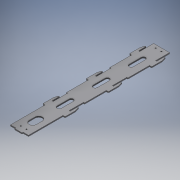
# Autodesk Inventor part: Camera mounting back
Saved by Autodesk Inventor 2017 (Build 210142000, 142)
## iProperties
Created: 2016-08-03
Part Number: Camera mounting back
Material: Generic
Document SubType Name: Modeling
Designer: Ali
Density: 1 g/cm^3
Appearance: Default
Author: Ali
Autodesk Inventor part; units mm, degrees
ref_plane "YZ Plane" through (0, 0, 0) normal (1, 0, 0) x (0, 1, 0)
ref_plane "XZ Plane" through (0, 0, 0) normal (0, 1, 0) x (-1, 0, 0)
ref_plane "XY Plane" through (0, 0, 0) normal (0, 0, 1) x (1, 0, 0)
sketch "Sketch1" plane through (0, 0, 0) normal (0, 0, 1) x (1, 0, 0)
  line L0 (-25, 0) -> (25, 0)
  line L1 (25, 0) -> (25, 394)
  line L2 (25, 394) -> (-25, 394)
  line L3 (-25, 394) -> (-25, 0)
  point P0 (0, 0)
  point P1 (0, 0)
  dimension "d0" = 394
  dimension "d1" = 50
  constraints: 8 end point, 3 perpendicular, 1 coincident, 1 horizontal, 1 midpoint
  measures "d0" distance of L0.end L1.end
  measures "d1" distance of L0.start L0.end
extrude "Extrusion1" add sketch "Sketch1" along normal blind 3
sketch "Sketch2" plane through (0, 0, 0) normal (0, 0, -1) x (-1, 0, 0)
  line L0 (-22, 334) -> (-25, 334)
  line L1 (-22, 374) -> (-25, 374)
  line L2 (-22, 374) -> (-22, 354)
  line L3 (-25, 334) -> (-25, 354)
  line L4 (-25, 0) -> (-25, 394) projected
  line L5 (-22, 354) -> (-25, 354)
  line L6 (-25, 0) -> (-25, 394) projected
  line L7 (-25, 394) -> (25, 394) projected
  line L8 (-25, 354) -> (-25, 374)
  line L9 (-22, 354) -> (-22, 334)
  line L10 (-22, 374) -> (-25, 374)
  line L11 (-25, 374) -> (-25, 394)
  line L12 (-25, 394) -> (-22, 394)
  line L13 (-22, 394) -> (-22, 374)
  point P0 (0, 0)
  dimension "d4" = 20
  dimension "d10" = 20
  dimension "d55" = 60
  dimension "d56" = 20
  constraints: 22 end point, 3 perpendicular, 3 point on line, 2 collinear, 2 parallel, 2 vertical, 1 horizontal
  measures "d4" distance between parallel lines of L1 L5
  measures "d10" distance of L12.end L1.start
  measures "d55" distance between parallel lines of L7 L0
  measures "d56" distance of L2.end L0.start
extrude "Extrusion2" cut sketch "Sketch2" against normal blind 3 contours L5 L4 L1 L2 | L1 L4 L7 L13
sketch "Sketch3" plane through (0, 0, 0) normal (0, 0, -1) x (-1, 0, 0)
  line L0 (-25, 0) -> (-25, 354) projected
  line L1 (-25, 354) -> (-31, 354)
  line L2 (-31, 354) -> (-31, 336)
  line L3 (-29, 334) -> (-25, 334)
  line L4 (-25, 334) -> (-25, 354)
  line L5 (-31, 354) -> (-25, 354)
  line L6 (-25, 354) -> (-25, 374)
  line L7 (-25, 374) -> (-28, 374)
  line L8 (-31, 364) -> (-31, 354)
  line L9 (-31, 364) -> (-28, 374)
  line L10 (-28, 374) -> (-31, 374) construction
  arc A0 (-31, 336) -> (-29, 334) centre (-29, 336) ccw
  point P0 (0, 0)
  point P1 (-31, 334)
  dimension "d11" = 20
  dimension "d12" = 20
  dimension "d13" = 6
  dimension "d16" = 2
  constraints: 20 end point, 5 parallel, 3 point on line, 2 horizontal, 2 perpendicular, 2 point on circle, 2 tangent, 1 centre point
  measures "d11" distance of L1.end point (-31, 334)
  measures "d12" distance of L10.end L1.end
  measures "d13" distance between parallel lines of L0 L2
  measures "d16" radius of A0
extrude "Extrusion3" add sketch "Sketch3" against normal blind 3
pattern_linear "Rectangular Pattern1" count 3 spacing 120 along (0, -1, 0) of "Extrusion2", "Extrusion3"
mirror "Mirror1" about plane through (0, 0, 0) normal (1, 0, 0) of "Extrusion2", "Rectangular Pattern1", "Extrusion3"
sketch "Sketch4" plane through (0, 0, 0) normal (0, 0, -1) x (-1, 0, 0)
  line L0 (-22, 384) -> (18.49, 384) construction
  line L1 (-22, 394) -> (22, 394) projected
  line L2 (-22, 394) -> (-22, 354) projected
  point P0 (0, 0)
  point P1 (-8, 384)
  point P2 (8, 384)
  dimension "d17" = 16
  dimension "d52" = 10
  dimension "d53" = 14
  constraints: 3 point on line, 2 end point, 1 horizontal
  measures "d17" distance of point (8, 384) point (-8, 384)
  measures "d52" distance between parallel lines of L1 L0
  measures "d53" distance from line of point (-8, 384) L2
hole "Hole1" at (8, 384, 0) at (-8, 384, 0) direction (0, 0, 1) diameter 3.2 end through all
sketch "Sketch5" plane through (0, 0, 0) normal (0, 0, -1) x (-1, 0, 0)
  line L0 (-10, 0) -> (10, 0)
  line L1 (-10, 0) -> (-10, -6)
  line L2 (10, -6) -> (-10, -6)
  line L3 (10, 0) -> (10, -6)
  line L4 (25, 94) -> (25, 0) projected
  point P0 (0, 0)
  dimension "d48" = 6
  dimension "d50" = 20
  dimension "d51" = 15
  constraints: 8 end point
  measures "d48" distance between parallel lines of L2 L0
  measures "d50" distance between parallel lines of L3 L1
  measures "d51" distance between parallel lines of L4 L3
extrude "Extrusion4" add sketch "Sketch5" against normal blind 3
sketch "Sketch6" plane through (0, 0, 0) normal (0, 0, -1) x (-1, 0, 0)
  line L0 (0, 36.6667) -> (0, 53.3333) construction
  line L1 (-10, 36.6667) -> (-10, 53.3333)
  line L2 (10, 53.3333) -> (10, 36.6667)
  arc A0 (-10, 36.6667) -> (10, 36.6667) centre (0, 36.6667) ccw
  arc A1 (10, 53.3333) -> (-10, 53.3333) centre (0, 53.3333) ccw
  line L3 (0, 343.6331) -> (0, 309.773) construction
  line L4 (-5.8349, 343.6331) -> (-5.8349, 309.773)
  line L5 (5.8349, 309.773) -> (5.8349, 343.6331)
  arc A2 (5.8349, 343.6331) -> (-5.8349, 343.6331) centre (0, 343.6331) ccw
  arc A3 (-5.8349, 309.773) -> (5.8349, 309.773) centre (0, 309.773) ccw
  line L6 (0, 243.6331) -> (0, 209.773) construction
  line L7 (-5.8349, 243.6331) -> (-5.8349, 209.773)
  line L8 (5.8349, 209.773) -> (5.8349, 243.6331)
  arc A4 (5.8349, 243.6331) -> (-5.8349, 243.6331) centre (0, 243.6331) ccw
  arc A5 (-5.8349, 209.773) -> (5.8349, 209.773) centre (0, 209.773) ccw
  line L9 (0, 143.6331) -> (0, 109.773) construction
  line L10 (-5.8349, 143.6331) -> (-5.8349, 109.773)
  line L11 (5.8349, 109.773) -> (5.8349, 143.6331)
  arc A6 (5.8349, 143.6331) -> (-5.8349, 143.6331) centre (0, 143.6331) ccw
  arc A7 (-5.8349, 109.773) -> (5.8349, 109.773) centre (0, 109.773) ccw
  point P0 (0, 0)
  point P1 (0, 45)
  point P2 (0, 326.7031)
  point P3 (0, 226.7031)
  point P4 (0, 126.7031)
  dimension "d28" = 10
  dimension "d29" = 45
  dimension "d43" = 100
  constraints: 32 end point, 16 point on circle, 8 centre point, 8 tangent, 3 vertical, 2 midpoint, 2 parallel, 1 collinear, 1 point on line, 23 other
  measures "d28" radius of A1
  measures "d29" distance of point (0, 0) point (0, 45)
  measures "d43" distance of L4.start L7.start
extrude "Extrusion5" cut sketch "Sketch6" against normal blind 3
sketch "Sketch7" plane through (0, 0, 0) normal (0, 0, -1) x (-1, 0, 0)
  line L0 (-22, 10) -> (26.4852, 10) construction
  line L1 (-25, 0) -> (-25, 94) projected
  line L2 (-10, 0) -> (-25, 0) projected
  point P0 (0, 0)
  point P1 (-8, 10)
  point P2 (8, 10)
  dimension "d32" = 16
  dimension "d33" = 17
  dimension "d54" = 10
  constraints: 2 end point, 2 point on line, 1 horizontal
  measures "d32" distance of point (8, 10) point (-8, 10)
  measures "d33" distance from line of L1 point (-8, 10)
  measures "d54" distance between parallel lines of L2 L0
hole "Hole2" at (8, 10, 0) at (-8, 10, 0) direction (0, 0, 1) diameter 3.2 end through all
body "Solid1"
